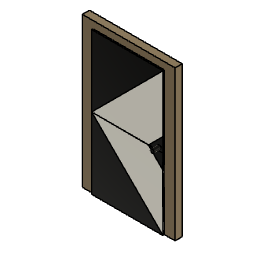
Evolution Door v2 (Autodesk Fusion 360 design; units mm, degrees)
Autodesk Fusion 360 part; units mm, degrees
sketch "Sketch1" plane through (0, 0, 0) normal (0, 1, 0) x (1, 0, 0) in component "BotLeft"
  line L0 (0, 0) -> (100, 0)
  line L1 (0, -100) -> (0, 0)
  line L2 (0, -100) -> (100, 0)
  line L3 (0, 0) -> (0, -3)
  line L4 (0, 0) -> (3, 0)
  circle A0 centre (3, -3) radius 1.5
  dimension "d1" = 100
  dimension "d2" = 100
  dimension "d38" = 3
  dimension "d39" = 3
  dimension "d40" = 3
  constraint horizontal L0
  constraint vertical L1
  constraint coincident L0.start L1.end
  constraint perpendicular L0 L3
  constraint perpendicular L1 L4
  measures "d1" distance of L0.start L0.end
  measures "d2" distance of L0.start L1.start
  measures "d38" distance of L0.start L3.end
  measures "d39" distance of L0.start L4.end
  measures "d40" diameter of A0
extrude "Extrude1" add sketch "Sketch1" against normal blind 2 contours L0 L1 L2 L3 L4 | A0 makes body 1 in component "BotLeft"
sketch "Sketch1 (2)" plane through (0, -2, 0) normal (0, -1, 0) x (1, 0, 0) in component "BotRight"
  line L0 (0, 100) -> (0, 0)
  line L1 (0, 0) -> (100, 0)
  line L2 (100, 0) -> (0, 100)
  line L3 (0, 100) -> (100, 100)
  line L4 (100, 100) -> (100, 0)
  line L5 (0, 100) -> (100, 0)
  line L6 (100, 100) -> (100, 80)
  line L7 (100, 100) -> (80, 100)
  line L8 (80, 100) -> (100, 80)
  dimension "d70" = 20
  dimension "d71" = 20
  constraint horizontal L3
  constraint vertical L4
  constraint coincident L1.end L2.start
  constraint coincident L0.start L2.end
  constraint perpendicular L3 L6
  constraint perpendicular L4 L7
  measures "d70" distance of L3.end L6.end
  measures "d71" distance of L3.end L7.end
extrude "Extrude1'" add sketch "Sketch1 (2)" against normal blind 2 separate body contours L2 L3 L4 L5 L8 | L3 L4 L6 L7 L8 makes body 2 in component "BotRight"
sketch "Sketch1 (3)" plane through (0, -2, 0) normal (0, -1, 0) x (1, 0, 0) in component "TopLeft"
  line L0 (0, 100) -> (0, 0)
  line L1 (0, 0) -> (100, 0)
  line L2 (100, 0) -> (0, 100)
  line L3 (100, 200) -> (0, 200)
  line L4 (0, 200) -> (0, 100)
  line L5 (0, 100) -> (100, 200)
  line L6 (0, 200) -> (0, 197)
  line L7 (0, 200) -> (3, 200)
  circle A0 centre (3, 197) radius 1.5
  dimension "d8" = 100
  dimension "d22" = 3
  dimension "d23" = 3
  dimension "d24" = 3
  constraint horizontal L3
  constraint vertical L4
  constraint coincident L0.start L2.end
  constraint perpendicular L3 L6
  constraint perpendicular L4 L7
  measures "d8" distance of L0.start L3.end
  measures "d22" distance of L3.end L6.end
  measures "d23" distance of L3.end L7.end
  measures "d24" diameter of A0
extrude "Extrude1''" add sketch "Sketch1 (3)" against normal blind 2 separate body contours L3 L4 L5 L6 L7 | A0 makes body 3 in component "TopLeft"
sketch "Sketch1 (4)" plane through (0, -2, 0) normal (0, -1, 0) x (1, 0, 0) in component "TopRight"
  line L0 (0, 100) -> (0, 0)
  line L1 (0, 0) -> (100, 0)
  line L2 (100, 0) -> (0, 100)
  line L3 (0, 100) -> (100, 200)
  line L4 (100, 200) -> (100, 100)
  line L5 (100, 100) -> (0, 100)
  line L6 (100, 100) -> (80, 100)
  line L7 (100, 100) -> (100, 120)
  line L8 (100, 120) -> (80, 100)
  dimension "d66" = 20
  dimension "d67" = 20
  constraint coincident L0.start L2.end
  constraint perpendicular L2 L3
  constraint parallel L0 L4
  constraint perpendicular L0 L5
  constraint perpendicular L4 L6
  constraint perpendicular L6 L7
  measures "d66" distance of L4.end L6.end
  measures "d67" distance of L4.end L7.end
extrude "Extrude1'''" add sketch "Sketch1 (4)" against normal blind 2 separate body contours L3 L4 L5 L8 | L4 L5 L6 L7 L8 makes body 4 in component "TopRight"
sketch "Sketch1 (5)" plane through (0, 0, 0) normal (0, 0, 1) x (1, 0, 0) in component "DoorFrame"
  line L0 (5, 0) -> (-15, 0)
  line L1 (-15, 0) -> (-15, 10)
  line L2 (-15, 10) -> (5, 10)
  line L3 (5, 10) -> (5, 0)
  line L4 (95, 0) -> (115, 0)
  line L5 (115, 0) -> (115, 10)
  line L6 (115, 10) -> (95, 10)
  line L7 (95, 10) -> (95, 0)
  dimension "d13" = 20
  dimension "d14" = 10
  dimension "d15" = 20
  dimension "d16" = 10
  constraint horizontal L0
  constraint vertical L1
  constraint horizontal L2
  constraint vertical L3
  constraint horizontal L4
  constraint vertical L5
  constraint horizontal L6
  constraint vertical L7
  measures "d13" distance of L0.start L0.end
  measures "d14" distance of L0.start L2.end
  measures "d15" distance of L4.start L4.end
  measures "d16" distance of L4.start L6.end
extrude "Extrude1''''" add sketch "Sketch1 (5)" along normal blind 210 separate body makes body 5 at (-1.6667, 0, 70) makes body 6 at (108.3333, 10, 70) in component "DoorFrame"
sketch "Sketch2" plane through (5, 0, 0) normal (1, 0, 0) x (0, 1, 0) in component "DoorFrame"
  line L0 (0, 0) -> (10, 0)
  line L1 (10, 0) -> (10, 210)
  line L2 (10, 210) -> (0, 210)
  line L3 (0, 210) -> (0, 0)
  line L4 (0, 200) -> (0, 195)
  line L5 (0, 195) -> (10, 195)
  dimension "d19" = 5
  constraint coincident L3 L4.start
  constraint coincident L1 L5.end
  constraint perpendicular L1 L5
  measures "d19" distance of L4.start L4.end
extrude "Extrude2" add sketch "Sketch2" along normal blind 90 contours L1 L2 L3 L4 L5 bodies 5 6 in component "DoorFrame"
extrude "Extrude2'" add sketch "Sketch1 (3)" against normal blind 8 contours A0 bodies 3 in component "TopLeft"
move_body "Move1" bodies 3 to x (1, 0, 0) y (0, 1, 0) z (0, 0, 1) at (0, -39, 0) in component "TopLeft"
sketch "Sketch3" plane through (0, 0, 0) normal (0, -1, 0) x (1, 0, 0) in component "DoorFrame"
  line L0 (-15, 0) -> (5, 0)
  line L1 (5, 0) -> (5, 195)
  line L2 (5, 195) -> (95, 195)
  line L3 (95, 195) -> (95, 0)
  line L4 (95, 0) -> (115, 0)
  line L5 (115, 0) -> (115, 210)
  line L6 (115, 210) -> (-15, 210)
  line L7 (-15, 210) -> (-15, 0)
  circle A0 centre (3, 197) radius 1.75
  dimension "d27" = 3.5
  measures "d27" diameter of A0
extrude "Extrude3" cut sketch "Sketch3" against normal blind 6 contours A0 bodies 5 in component "DoorFrame"
extrude "Extrude2''" add sketch "Sketch1" along normal blind 8 contours A0 bodies 1 in component "BotLeft"
sketch "Sketch4" plane through (0, 0, 0) normal (0, -1, 0) x (1, 0, 0) in component "DoorFrame"
  circle A0 centre (3, 197) radius 1.75
  line L0 (-15, 0) -> (5, 0)
  line L1 (5, 0) -> (5, 195)
  line L2 (5, 195) -> (95, 195)
  line L3 (95, 195) -> (95, 0)
  line L4 (95, 0) -> (115, 0)
  line L5 (115, 0) -> (115, 210)
  line L6 (115, 210) -> (-15, 210)
  line L7 (-15, 210) -> (-15, 0)
  circle A1 centre (3, 3) radius 1.75
  dimension "d43" = 3.5
  measures "d43" diameter of A1
extrude "Extrude4" cut sketch "Sketch4" against normal blind 8 contours A1 bodies 5 in component "DoorFrame"
move_body "Move1'" bodies 1 to x (1, 0, 0) y (0, 1, 0) z (0, 0, 1) at (0, -18, 0) in component "BotLeft"
move_body "Move1''" bodies 4 to x (1, 0, 0) y (0, 1, 0) z (0, 0, 1) at (0, -40, 0) in component "TopRight"
move_body "Move1'''" bodies 2 to x (1, 0, 0) y (0, 1, 0) z (0, 0, 1) at (0, -40, 0) in component "BotRight"
extrude "Extrude2'''" cut sketch "Sketch1 (4)" along normal blind 43 contours L4 L5 L6 L7 L8 bodies 4 in component "TopRight"
extrude "Extrude2''''" cut sketch "Sketch1 (2)" along normal blind 56 contours L3 L4 L6 L7 L8 bodies 2 in component "BotRight"
move_body "Move2" bodies 2 to x (1, 0, 0) y (0, 1, 0) z (0, 0, 1) at (0, 40, 0) in component "BotRight"
move_body "Move2'" bodies 4 to x (1, 0, 0) y (0, 1, 0) z (0, 0, 1) at (0, 40, 0) in component "TopRight"
sketch "Sketch1 (6)" plane through (0, -2, 0) normal (0, -1, 0) x (1, 0, 0) in component "TopSmall"
  line L0 (-0.0417, 99.9987) -> (0.0013, -0.0013)
  line L1 (0.0013, -0.0013) -> (100.0013, 0.0417)
  line L2 (100.0013, 0.0417) -> (-0.0417, 99.9987)
  line L3 (80, 100) -> (100, 100)
  line L4 (100, 100) -> (100, 120)
  line L5 (100, 120) -> (80, 100)
  line L6 (100, 100) -> (95.0503, 104.9497)
  line L7 (100, 100) -> (93, 100) construction
  circle A0 centre (95.0503, 104.9497) radius 2.5
  dimension "d90" = 45
  dimension "d91" = 7
  dimension "d92" = 5
  constraint horizontal L3
  constraint perpendicular L3 L4
  constraint horizontal L7
  constraint coincident L6.end A0.centre
  measures "d90" angle of L6 L7
  measures "d91" distance of L3.end L6.end
  measures "d92" diameter of A0
extrude "Extrude1'''''" add sketch "Sketch1 (6)" against normal blind 2 separate body contours L3 L4 L5 | A0 makes body 7 in component "TopSmall"
sketch "Sketch1 (7)" plane through (0, -2, 0) normal (0, -1, 0) x (1, 0, 0) in component "BotSmall"
  line L0 (-0.0417, 99.9987) -> (0.0013, -0.0013)
  line L1 (0.0013, -0.0013) -> (100.0013, 0.0417)
  line L2 (100.0013, 0.0417) -> (-0.0417, 99.9987)
  line L3 (100, 100) -> (100, 80)
  line L4 (100, 80) -> (80, 100)
  line L5 (80, 100) -> (100, 100)
  constraint vertical L3
  constraint perpendicular L3 L5
extrude "Extrude1''''''" add sketch "Sketch1 (7)" against normal blind 2 separate body contours L3 L4 L5 makes body 8 in component "BotSmall"
extrude "Extrude2'''''" add sketch "Sketch1 (6)" along normal blind 10 contours A0 bodies 7 in component "TopSmall"
component "TopLeft" placed x (0.995873, 0, -0.090754) y (0, 1, 0) z (0.090754, 0, 0.995873) at (-17.8662, 39, 1.0852)
component "TopRight" placed x (0.995873, 0, -0.090754) y (0, 1, 0) z (0.090754, 0, 0.995873) at (-17.8662, 0, 1.0852)
component "BotRight" placed x (0.994165, -0.107647, 0.006991) y (0.10625, 0.988344, 0.109026) z (-0.018646, -0.107647, 0.994014) at (0.8267, 10.7414, 0.7699)
component "BotLeft" placed x (0.999917, 0, 0.012894) y (0, 1, 0) z (-0.012894, 0, 0.999917) at (0.0389, 18, -0.0384)
component "DoorFrame" placed x (1, 0, 0) y (0, 1, 0) z (0, 0, 1) at (0, 0, 0)
component "TopSmall" placed x (0.962342, 0.267112, -0.050498) y (-0.241768, 0.925906, 0.290251) z (0.124286, -0.267112, 0.955617) at (-18.5368, 5.3422, 1.8903)
component "BotSmall" placed x (-0.431275, 0.698865, 0.570604) y (0.689796, -0.152236, 0.707818) z (0.581535, 0.698865, -0.416418) at (76.4795, -134.7352, 78.3993)
equation "d90 = 0 deg + 45 deg"
